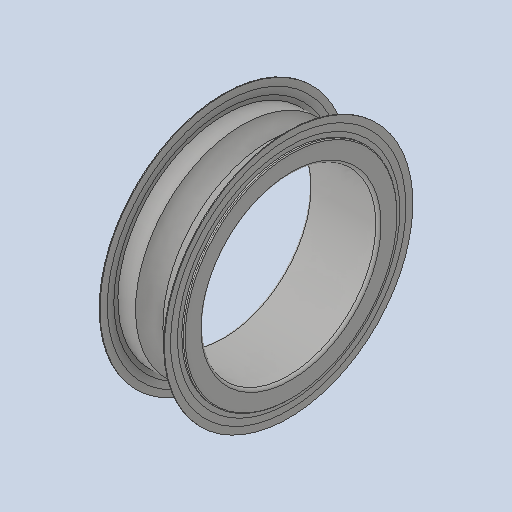
# Autodesk Inventor part: SKF_W 61700 X-2RS1_PART1
Saved by Autodesk Inventor 2022 (Build 260153000, 153)
## iProperties
Created: 2022-07-30
Part Number: SKF_W 61700 X-2RS1_PART1
Material: Generic
Catalog Web Link: www.cadenas.de
Description: -Deep groove ball bearings
Vendor: SKF
Document SubType Name: Modeling
Designer: psAdmin
Manufacturer: SKF
Mass: 2 g
Surface Area: 5.33348 cm^2
Volume: 0.131515 cm^3
Density: 1 g/cm^3
Appearance: PSOLRGB-175-175-175
Category: PARTsolutions
Company: SKF
PSOL_IDENT_0: {$CADENAS_DATA/23d-libs/skf/bearings_units_and_housings/ball_bearings/deep_groove_ball_bearings/bb1_
PSOL_IDENT_1: 001_101.prj},215 {VTYP=3D},{NB=SKF_W 61700 X-2RS1_PART1},{LINA=SKF_W 61700 X-2RS1_PART1},{NN=BB1_001
PSOL_IDENT_2: _101_PART1},{NOPRJ=TRUE},{DATE=29.07.2022 12:16:16},{GEOMDATE=04.07.2022 10:54:51},{VERSION=},{LINEI
PSOL_IDENT_3: D=18530},{WBVAR=},{WBNUMERIC=}  {NB=SKF_W 61700 X-2RS1_PART1},{LINA=SKF_W 61700 X-2RS1_PART1},{KT=DU
PSOL_IDENT_4: MMY},{DESIGNATION=W 61700 X-2RS1},{R12=0.15},{DD=10.000},{D=15.000},{B=4.000},{C=},{CX=},{CXX=},{CA=
PSOL_IDENT_5: 0.000},{XXVARIANT=},{XXDESIGN=Single row stainless steel},{XXSEALING=Contact seal on both sides},{DE
PSOL_IDENT_6: SIGN=dgbbw2rs},{DESIGNIR=dgbbw2rs},{VARIANT=},{DD1=11.21},{DD2=11.21},{DD2X=},{DD2A=11.21},{D1=13.60
PSOL_IDENT_7: },{D1X=0.00},{D2=14.2},{D2A=14.20},{D3=},{D3X=},{D3A=0.000},{D4=},{HH=0.000},{BB=0.000},{BBX=},{BBA=
PSOL_IDENT_8: 0.000},{FF=},{R0MAX=0.000},{R0=0.000},{PITCH=12.49},{DW=1.588},{DDAMIN=11.000},{DDAMAX=11.000},{DDBM
PSOL_IDENT_9: IN=0.000},{DDBMAX=0.000},{DBMIN=0.000},{DAMAX=14.500},{BBAMIN=0.000},{CAMAX=0.000},{RAMAX=0.150},{LO
PSOL_IDENT_10: AD1=0.488},{LOAD2=0.220},{LOAD3=0.009},{SPEED1=0},{SPEED2=24000},{KR=0.015},{F0=8.000},{Z=11},{II=1}
PSOL_IDENT_11: ,{MASS=0.002},{BEARING=W 61700 X-2RS1},{RING=},{HELP=0.700},{HELP2=0.400},{DD1ALG=5.605},{YALG=5.605
PSOL_IDENT_12: },{PITCH1=12.490},{DW1=1.588},{YALG1=6.800},{HALG1=0.700},{SH=5.605},{CU=0.482},{HALG=0.605},{B1=0},
PSOL_IDENT_13: {SHIELDHELP=2},{D4A=0.000},{FFA=0.000},{RS1=},{HELP3=0}
NB: SKF_W 61700 X-2RS1_PART1
NT: Deep groove ball bearings
NBSYN: SKF_$DESIGNATION._PART1
LINA: SKF_W 61700 X-2RS1_PART1
CATALOG: SKF
DESIGNATION: W 61700 X-2RS1
R12: 0.15
DD: 10
D: 15
B: 4
XXDESIGN: Single row stainless steel
XXSEALING: Contact seal on both sides
DD2: 11.21
D2: 14.2
LOAD1: 0.488
LOAD2: 0.22
LOAD3: 0.009
SPEED1: 0
SPEED2: 24000
BEARING: W 61700 X-2RS1
SUPPLIER: SKF
ARTICLENO: SKF_W 61700 X-2RS1_PART1
BOMINFO: SKF_W 61700 X-2RS1_PART1
CREATOR: CADENAS GmbH
Title: SKF_W 61700 X-2RS1_PART1
Author: Cadenas PARTsolutions
Comments: Deep groove ball bearings
Autodesk Inventor part; units mm, degrees
ref_plane "YZ Plane" through (0, 0, 0) normal (1, 0, 0) x (0, 1, 0)
ref_plane "XZ Plane" through (0, 0, 0) normal (0, 1, 0) x (-1, 0, 0)
ref_plane "XY Plane" through (0, 0, 0) normal (0, 0, 1) x (1, 0, 0)
sketch "Sketch_13" plane through (0, 0, 0) normal (0, 0, 1) x (1, 0, 0)
  line L0 (50, 0) -> (-50, 0)
  line L1 (0, 6.055) -> (0, 5.15)
  arc A0 (0, 5.15) -> (0.15, 5) centre (0.15, 5.15) ccw
  line L2 (0.15, 5) -> (3.85, 5)
  arc A1 (3.85, 5) -> (4, 5.15) centre (3.85, 5.15) ccw
  line L3 (4, 5.15) -> (4, 6.055)
  arc A2 (4, 6.055) -> (3.95, 6.105) centre (3.95, 6.055) ccw
  line L4 (3.95, 6.105) -> (2.7816, 6.105)
  arc A3 (1.2184, 6.105) -> (2.7816, 6.105) centre (2, 6.245) ccw
  line L5 (1.2184, 6.105) -> (0.05, 6.105)
  arc A4 (0.05, 6.105) -> (0, 6.055) centre (0.05, 6.055) ccw
  constraints: 12 end point, 10 point on circle, 5 centre point
revolve "Revolution1" add sketch "Sketch_13" angle 360 about axis through (50, 0, 0) along (1, 0, 0)
sketch "Sketch_15" plane through (0, 0, 0) normal (0, 0, 1) x (1, 0, 0)
  line L0 (50, 0) -> (-50, 0)
  line L1 (0.135, 7.1) -> (0.1575, 6.7263)
  line L2 (0.1575, 6.7263) -> (0.135, 6.3525)
  line L3 (0.135, 6.3525) -> (0.135, 5.605)
  line L4 (0.135, 5.605) -> (0.18, 5.605)
  line L5 (0.18, 5.605) -> (0.225, 6.3525)
  line L6 (0.225, 6.3525) -> (0.225, 6.7263)
  line L7 (0.225, 6.7263) -> (0.18, 7.1)
  line L8 (0.18, 7.1) -> (0.135, 7.1)
  constraints: 18 end point
revolve "Revolution2" add sketch "Sketch_15" angle 360 about axis through (50, 0, 0) along (1, 0, 0)
sketch "Sketch_16" plane through (0, 0, 0) normal (0, 0, 1) x (1, 0, 0)
  line L0 (50, 0) -> (-50, 0)
  line L1 (3.775, 6.7263) -> (3.775, 6.3525)
  line L2 (3.775, 6.3525) -> (3.82, 5.605)
  line L3 (3.82, 5.605) -> (3.865, 5.605)
  line L4 (3.865, 5.605) -> (3.865, 6.3525)
  line L5 (3.865, 6.3525) -> (3.8425, 6.7263)
  line L6 (3.8425, 6.7263) -> (3.865, 7.1)
  line L7 (3.865, 7.1) -> (3.82, 7.1)
  line L8 (3.82, 7.1) -> (3.775, 6.7263)
  constraints: 18 end point
revolve "Revolution3" add sketch "Sketch_16" angle 360 about axis through (50, 0, 0) along (1, 0, 0)
body "Solid1"
